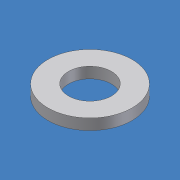
# Autodesk Inventor part: HCBST5washer2
Saved by Autodesk Inventor 2014 SP1 (Build 180222100, 222)
## iProperties
Category: PARTsolutions
Created: 2015-02-04
Part Number: HCBST5washer2
Catalog Web Link: www.cadenas.de
Description: HCBSTw2 - Washer Assembled Hexagon Socket Head Cap Screws
Document SubType Name: Modeling
Designer: PARTsolutions
Material: Generic
Density: 1 g/cm^3
Appearance: RGB(192,192,192)
NB: HCBST5washer2
NN: HCBSTw2
NT: Washer Assembled Hexagon Socket Head Cap Screws
NBSYN: $PN.washer2
LINA: HCBST5
PN: HCBST5
M: 5
M1: 5
MP: 5x0.8
P: 0.800
C: 8.5
D: 10.0
AA: 5.4
DD: 5.1
TT: 1.3
KT: DUMMY
SUPPLIER: Misumi
ARTICLENO: HCBST5washer2
BOMINFO: HCBST5
CREATOR: CADENAS GmbH
PSOL_IDENT_0: {\\10.0.0.236\data_v8\23d-libs\misumi\metric\38_al_extrusions_blackets\nuts\hcbst_washer.prj},162 {V
PSOL_IDENT_1: TYP=3D},{NB=HCBST5washer2},{LINA=HCBST5},{NN=HCBSTw2},{DATE=19.11.2014 02:34:01},{GEOMDATE=18.08.200
PSOL_IDENT_2: 9 10:36:00},{VERSION=},{LINEID=40},{LINESUBID=-1},{WBVAR=}  {NB=HCBST5washer2},{LINA=HCBST5},{KT=DUM
PSOL_IDENT_3: MY},{PN=HCBST5},{M=5},{M1=5},{MP=5x0.8},{P=0.800},{C=8.5},{D=10.0},{AA=5.4},{DD=5.1},{TT=1.3}
Title: HCBST5
Author: Cadenas PARTsolutions
Comments: Washer Assembled Hexagon Socket Head Cap Screws
Autodesk Inventor part; units mm, degrees
sketch "Sketch_2" plane through (0, 0, 0) normal (0, 0, 1) x (1, 0, 0)
  circle A0 centre (0, 0) radius 5
  circle A1 centre (0, 0) radius 2.55
  constraints: 2 centre point
extrude "Extrusion1" add sketch "Sketch_2" against normal blind 1.3
ref_plane "washer_to_bolt_XY" through (0, 0, 0) normal (0, 0, 1) x (1, 0, 0)
ref_plane "washer_to_bolt_YZ" through (0, 0, 0) normal (1, 0, 0) x (0, 1, 0)
ref_plane "washer_to_bolt_ZX" through (0, 0, 0) normal (0, 1, 0) x (0, 0, 1)
body "Solid1"
